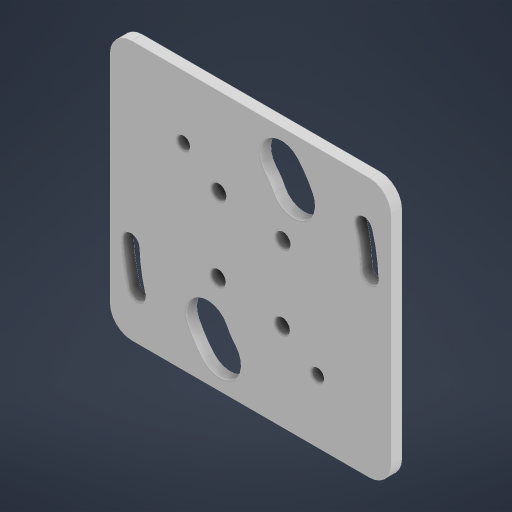
# Autodesk Inventor part: mount-plate
Saved by Autodesk Inventor 2024 (Build 280153000, 153)
## iProperties
Created: 2024-05-17
Part Number: mount-plate
Material: Generic
Document SubType Name: Modeling
Designer: loren
Density: 1 g/cm^3
Appearance: Default
Author: loren
## iProperties of the stored document mount-plate_3DPrint.ipt
Created: 2026-02-06
Part Number: mount-plate_3DPrint
Material: Generic
Document SubType Name: Modeling
Designer: lokies
Density: 1 g/cm^3
Appearance: Default
Author: lokies
Autodesk Inventor part; units mm, degrees
ref_plane "YZ Plane" through (0, 0, 0) normal (1, 0, 0) x (0, 1, 0)
ref_plane "XZ Plane" through (0, 0, 0) normal (0, 1, 0) x (-1, 0, 0)
ref_plane "XY Plane" through (0, 0, 0) normal (0, 0, 1) x (1, 0, 0)
sketch "Sketch1" plane through (0, 0, 0) normal (0, 0, 1) x (1, 0, 0)
  line L0 (-32.5, 30) -> (32.5, 30)
  line L1 (32.5, 30) -> (32.5, -30)
  line L2 (32.5, -30) -> (-32.5, -30)
  line L3 (-32.5, -30) -> (-32.5, 30)
  point P0 (0, 0)
  point P1 (32.5, 0)
  point P2 (0, 30)
  dimension "d31" = 65
  dimension "d32" = 60
  constraints: 8 end point, 2 midpoint, 2 parallel, 1 horizontal, 1 horizontal alignment, 1 perpendicular, 1 vertical alignment
  measures "d31" distance of L0.start L0.end
  measures "d32" distance of L0.end L1.end
extrude "Extrusion1" add sketch "Sketch1" along normal blind 2.5
sketch "Sketch2" plane through (0, 0, 2.5) normal (0, 0, 1) x (1, 0, 0)
  circle A0 centre (-15.5, 15.5) radius 1.5
  line L0 (-15.5, 15.5) -> (9.1537, 19.6464) construction
  line L1 (9.1537, 19.6464) -> (10.0481, 11.6966) construction
  line L2 (-7.3422, 9.7403) -> (27.4384, 13.6529) construction
  circle A1 centre (10.0481, 11.6966) radius 14 construction
  line L3 (4.1293, -0.9907) -> (4.6943, -6.0129)
  line L4 (4.6943, -6.0129) -> (19.2027, -4.3808) construction
  line L5 (19.2027, -4.3808) -> (18.6378, 0.6414)
  circle A2 centre (-15.5, 15.5) radius 19.9154 construction
  circle A3 centre (9.1537, 19.6464) radius 7.5 construction
  line L6 (-15.5, 15.5) -> (15.5, -15.5) construction
  circle A4 centre (15.5, -15.5) radius 19.9154 construction
  line L7 (-18.6378, -0.6414) -> (-19.2027, 4.3808)
  line L8 (18.9203, -1.8697) -> (-18.9203, 1.8697) construction
  line L9 (-4.1293, 0.9907) -> (-4.6943, 6.0129)
  line L10 (4.4118, -3.5018) -> (-4.4118, 3.5018) construction
  arc A5 (25.6476, 10.5572) -> (24.3121, 19.0678) centre (-7.3422, 9.7403) ccw
  arc A6 (25.6476, 10.5572) -> (29.6464, 10.6562) centre (27.647, 10.6067) ccw
  arc A7 (29.6464, 10.6562) -> (28.149, 20.1984) centre (-7.3422, 9.7403) ccw
  arc A8 (28.149, 20.1984) -> (24.3121, 19.0678) centre (26.2305, 19.6331) ccw
  arc A9 (27.647, 10.6067) -> (26.2305, 19.6331) centre (-7.3422, 9.7403) ccw construction
  arc A10 (9.9544, 18.171) -> (7.1829, 22.3604) centre (-7.3422, 9.7403) ccw construction
  arc A11 (5.4598, 15.9803) -> (3.4086, 19.0811) centre (-7.3422, 9.7403) ccw
  arc A12 (10.9573, 25.6398) -> (3.4086, 19.0811) centre (7.1829, 22.3604) ccw
  arc A13 (14.4489, 20.3618) -> (10.9573, 25.6398) centre (-7.3422, 9.7403) ccw
  arc A14 (5.4598, 15.9803) -> (14.4489, 20.3618) centre (9.9544, 18.171) ccw
  circle A15 centre (-7.3422, 9.7403) radius 1.75
  circle A16 centre (7.5, 7.5) radius 1.75
  line L11 (0, 0) -> (7.5, 7.5) construction
  line L12 (-4.6943, 6.0129) -> (-3.0147, 6.6604) construction
  circle A17 centre (9.9544, 18.171) radius 7.5
  circle A18 centre (0, 0) radius 13.25
  dimension "d3" = 15.5
  dimension "d4" = 3
  dimension "d5" = 15.5
  dimension "d6" = 25
  dimension "d7" = 8
  dimension "d8" = 35
  dimension "d9" = 28
  dimension "d11" = 17
  dimension "d12" = 14.6
  dimension "d13" = 39.8307
  dimension "d14" = 15
  dimension "d17" = 4
  dimension "d18" = 5
  dimension "d19" = 10
  dimension "d20" = 5
  dimension "d21" = 10
  dimension "d22" = 10
  dimension "d23" = 3.5
  dimension "d27" = 7.5
  dimension "d35" = 4
  dimension "d36" = 1.8
  dimension "d37" = 15
  dimension "d38" = 26.5
  constraints: 26 end point, 25 point on circle, 19 centre point, 16 coincident, 8 midpoint, 8 tangent, 6 parallel, 4 perpendicular, 2 equal radius, 1 line through centre
  measures "d3" horizontal distance of point (0, 0) L0.start
  measures "d4" diameter of A0
  measures "d5" horizontal distance of point (0, 0) L0.start
  measures "d6" distance of L0.start L0.end
  measures "d7" distance of L0.end L1.end
  measures "d8" distance of L2.start L2.end
  measures "d9" diameter of A1
  measures "d11" distance from line of L1.end L4
  measures "d12" distance of L3.end L4.end
  measures "d13" diameter of A2
  measures "d14" diameter of A3
  measures "d17" radial gap between concentric circles of A7 A5
  measures "d22" radial gap between concentric circles of A11 A13
  measures "d23" diameter of A15
  measures "d27" horizontal distance of point (0, 0) L11.end
  measures "d35" distance from line of L9.end L2
  measures "d36" distance of L9.end L12.end
  measures "d37" diameter of A17
  measures "d38" diameter of A18
extrude "Extrusion2" cut sketch "Sketch2" against normal blind 3 contours A0 | A5 A8 A7 A6 | A11 A12 A17 A13 A14 | A12 A13 A17 | A18 A15 | A15 A18 | A16
pattern_circular "Circular Pattern1" count 2 over 360 about axis through (0, 0, -10) along (0, 0, 1) of "Extrusion2"
fillet "Fillet1" radius 5 4 edges at (32.5, 30, 1.25) (32.5, -30, 1.25) (-32.5, -30, 1.25) (-32.5, 30, 1.25)
equation "\"d3\" = 0.5 * mount_screw_ortho_dist"
equation "\"d4\" = screw_dia"
equation "\"d5\" = d3"
equation "\"d7\" = stepper_axis_offset"
equation "\"d8\" = stepper_screw_dist"
equation "\"d9\" = stepper_dia"
equation "\"d13\" = HeadDiameter"
equation "\"stepper_screw_dist\" = 35"
equation "\"stepper_axis_offset\" = 8"
equation "\"mount_screw_ortho_dist\" = 31"
equation "\"screw_dia\" = 3"
equation "\"stepper_dia\" = 28"
equation "\"thumbscrew_dia\" = 15.8"
equation "\"helix_length\" = 3.5"
equation "\"helix_width\" = 2"
equation "\"helix_fillet\" = 0.3"
equation "\"helix_inner_dia\" = 19"
equation "\"helix_outer_dia\" = 23"
equation "\"elephant_prevention_radius\" = 0.3"
equation "\"gear_center_distance\" = 25"
equation "\"sheet_thick\" = 2.5"
equation "\"helix_winding_factor\" = 1.2"
equation "\"HeadDiameter\" = 39.830729"
body "Solid1"
